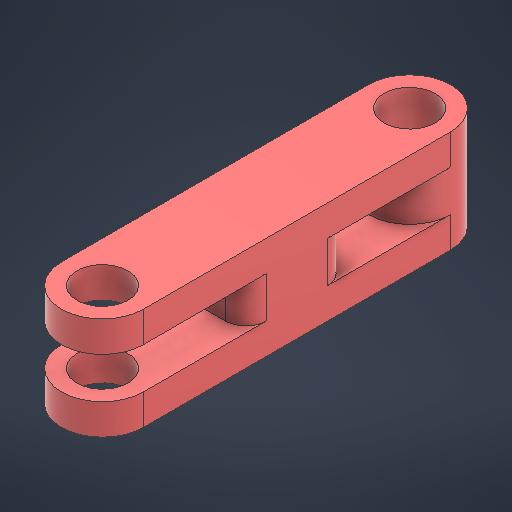
# Autodesk Inventor part: connector
Saved by Autodesk Inventor 2027 (Build 310192060, 192F)
## iProperties
Created: 2026-08-20
Part Number: connector
Material: Ogólny
Document SubType Name: Modeling
Designer: User
Density: 1 g/cm^3
Appearance: Domyślna
Author: User
Autodesk Inventor part; units mm, degrees
ref_plane "YZ Plane" through (0, 0, 0) normal (1, 0, 0) x (0, 1, 0)
ref_plane "XZ Plane" through (0, 0, 0) normal (0, 1, 0) x (-1, 0, 0)
ref_plane "XY Plane" through (0, 0, 0) normal (0, 0, 1) x (1, 0, 0)
sketch "Szkic1" plane through (0, 0, 0) normal (0, 1, 0) x (-1, 0, 0)
  line L0 (0, 15) -> (0, -15) construction
  line L1 (-4, 15) -> (-4, -15)
  line L2 (4, -15) -> (4, 15)
  arc A0 (4, 15) -> (-4, 15) centre (0, 15) ccw
  arc A1 (-4, -15) -> (4, -15) centre (0, -15) ccw
  circle A2 centre (0, -15) radius 2.5
  circle A3 centre (0, 15) radius 2.5
  line L3 (0, 15) -> (0, 5)
  line L4 (0, 5) -> (4, 5)
  line L5 (0, 5) -> (-4, 5)
  point P0 (0, 0)
  dimension "d0" = 15
  dimension "d1" = 8
  dimension "d2" = 5
  dimension "d3" = 5
  dimension "d6" = 10
  constraints: 14 end point, 4 centre point, 4 point on circle, 4 point on line, 4 tangent, 2 coincident, 1 midpoint, 1 parallel, 1 perpendicular, 1 vertical
  measures "d0" distance of point (0, 0) L0.end
  measures "d1" diameter of A1
  measures "d2" diameter of A2
  measures "d3" diameter of A3
  measures "d6" distance of L3.start L3.end
extrude "Wyciągnięcie proste1" add sketch "Szkic1" along normal mid plane 10 contours A0 L2 L4 L5 L1 | L5 L4 L2 A1 L1 | A2 | A3
extrude "Wyciągnięcie proste2" cut sketch "Szkic1" along normal mid plane 4 contours A0 L2 L4 L5 L1
extrude "Wyciągnięcie proste3" cut sketch "Szkic1" along normal mid plane 14.5 contours A3
mirror "Odbij1" about plane through (0, 0, 0) normal (0, 0, 1) of "Wyciągnięcie proste2", "Wyciągnięcie proste3"
fillet "Zaokrąglenie1" radius 2 4 edges at (-4, 0, 5) (-4, 0, -5) (4, 0, -5) (4, 0, 5)
sketch "Szkic2" plane through (0, 5, 0) normal (0, 1, 0) x (1, 0, 0)
  circle A0 centre (0, 15) radius 2.5 projected
  circle A1 centre (0, 15) radius 4
  circle A2 centre (0, 15) radius 2.5
  point P0 (0, 0)
  constraints: 2 centre point, 2 coincident, 1 concentric
extrude "Wyciągnięcie proste4" add sketch "Szkic2" against normal up to surface (10 mm away)
